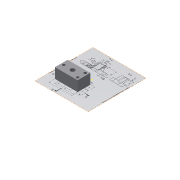
# Autodesk Inventor part: Основание
Saved by Autodesk Inventor 2014 SP1 (Build 180222100, 222)
## iProperties
Created: 2023-10-15
Part Number: Основание
Material: Типовые
Document SubType Name: Modeling
Designer: Konstantin
Density: 1 g/cm^3
Appearance: По умолчанию
Author: Konstantin
Autodesk Inventor part; units mm, degrees
ref_plane "YZ Plane" through (0, 0, 0) normal (1, 0, 0) x (0, 1, 0)
ref_plane "XZ Plane" through (0, 0, 0) normal (0, 1, 0) x (-1, 0, 0)
ref_plane "XY Plane" through (0, 0, 0) normal (0, 0, 1) x (1, 0, 0)
sketch "Эскиз1" plane through (0, 0, 0) normal (0, 0, 1) x (1, 0, 0)
  line L0 (-109.4005, 113.4321) -> (101.5019, 113.4321) construction
  line L1 (101.5019, 113.4321) -> (101.5019, -116.5229) construction
  line L2 (101.5019, -116.5229) -> (-109.4005, -116.5229) construction
  line L3 (-109.4005, -116.5229) -> (-109.4005, 113.4321) construction
  point P0 (0, 0)
  constraints: 2 other
sketch "Эскиз3" plane through (0, 0, 0) normal (0, 0, 1) x (1, 0, 0)
  line L0 (13.0914, -19.0842) -> (-76.7694, -19.0842)
  line L1 (-76.7694, -19.0842) -> (-76.7694, -69.3185)
  line L2 (-76.7694, -69.3185) -> (13.0914, -69.3185)
  line L3 (13.0914, -69.3185) -> (13.0914, -19.0842)
  circle A0 centre (-31.9077, -44.3035) radius 8.6947
  circle A1 centre (-31.9077, -44.3035) radius 14.858
  circle A2 centre (-66.8024, -44.2775) radius 5.0913
  circle A3 centre (3.2723, -59.1355) radius 4.9697
  circle A4 centre (3.2723, -29.4194) radius 5.2903
  line L4 (-61.7111, -29.3433) -> (-64.4086, -29.3433) construction
  line L5 (-64.4086, -29.3433) -> (-66.8024, -30.0442) construction
  line L6 (-66.8024, -30.0442) -> (-70.0469, -31.5698) construction
  line L7 (-70.0469, -31.5698) -> (-73.0319, -33.7588) construction
  line L8 (-73.0319, -33.7588) -> (-75.0219, -36.9428) construction
  line L9 (-75.0219, -36.9428) -> (-76.7694, -40.6575) construction
  line L10 (-76.7694, -40.6575) -> (-76.7694, -44.2013) construction
  line L11 (-76.7694, -44.2013) -> (-76.7694, -47.6888) construction
  line L12 (-76.7694, -47.6888) -> (-75.1545, -51.4698) construction
  line L13 (-75.1545, -51.4698) -> (-72.7665, -54.9191) construction
  line L14 (-72.7665, -54.9191) -> (-69.2509, -57.5061) construction
  line L15 (-69.2509, -57.5061) -> (-66.4649, -58.7001) construction
  line L16 (-66.4649, -58.7001) -> (-63.4136, -59.0593) construction
  line L17 (-63.4136, -59.0593) -> (-61.7111, -59.5624) construction
  spline S0 degree 4 poles (-61.7111, -29.3433) (-64.4086, -29.3433) (-66.8024, -30.0442) (-70.0469, -31.5698) (-73.0319, -33.7588) (-75.0219, -36.9428) (-76.7694, -40.6575) (-76.7694, -44.2013) (-76.7694, -47.6888) (-75.1545, -51.4698) (-72.7665, -54.9191) (-69.2509, -57.5061) (-66.4649, -58.7001) (-63.4136, -59.0593) (-61.7111, -59.5624) knots 1 1 1 1 1 2 3 4 5 6 7 8 9 10 11 12 12 12 12 12
  line L18 (-61.7111, -59.5624) -> (-61.7111, -74.6864)
  line L19 (-61.7111, -29.3433) -> (-61.7111, -13.2619)
  line L20 (-61.7111, -13.2619) -> (-82.7829, -13.2619)
  line L21 (-82.7829, -13.2619) -> (-82.7829, -74.6864)
  line L22 (-82.7829, -74.6864) -> (-61.7111, -74.6864)
  line L23 (0.9069, -17.4974) -> (3.1443, -19.2421) construction
  line L24 (3.1443, -19.2421) -> (3.2723, -19.427) construction
  line L25 (3.2723, -19.427) -> (4.9671, -19.427) construction
  line L26 (4.9671, -19.427) -> (6.9505, -20.1638) construction
  line L27 (6.9505, -20.1638) -> (8.5626, -20.9222) construction
  line L28 (8.5626, -20.9222) -> (10.1498, -22.3051) construction
  line L29 (10.1498, -22.3051) -> (11.3609, -23.7137) construction
  line L30 (11.3609, -23.7137) -> (12.2956, -25.2934) construction
  line L31 (12.2956, -25.2934) -> (13.0914, -26.9858) construction
  line L32 (13.0914, -26.9858) -> (16.1389, -44.0503) construction
  line L33 (16.1389, -44.0503) -> (13.0914, -59.6386) construction
  line L34 (13.0914, -59.6386) -> (13.0914, -61.2275) construction
  line L35 (13.0914, -61.2275) -> (12.4731, -63.3199) construction
  line L36 (12.4731, -63.3199) -> (11.3461, -64.8514) construction
  line L37 (11.3461, -64.8514) -> (10.2973, -66.2768) construction
  line L38 (10.2973, -66.2768) -> (8.7533, -67.6316) construction
  line L39 (8.7533, -67.6316) -> (7.3634, -68.5939) construction
  line L40 (7.3634, -68.5939) -> (4.8885, -69.3185) construction
  line L41 (4.8885, -69.3185) -> (3.2723, -70.0088) construction
  line L42 (3.2723, -70.0088) -> (2.887, -71.3126) construction
  line L43 (2.887, -71.3126) -> (31.3831, -71.3126) construction
  line L44 (31.3831, -71.3126) -> (20.1564, -15.836) construction
  line L45 (20.1564, -15.836) -> (1.0706, -16.7541) construction
  spline S1 degree 4 poles (0.9069, -17.4974) (3.1443, -19.2421) (3.2723, -19.427) (4.9671, -19.427) (6.9505, -20.1638) (8.5626, -20.9222) (10.1498, -22.3051) (11.3609, -23.7137) (12.2956, -25.2934) (13.0914, -26.9858) (16.1389, -44.0503) (13.0914, -59.6386) (13.0914, -61.2275) (12.4731, -63.3199) (11.3461, -64.8514) (10.2973, -66.2768) (8.7533, -67.6316) (7.3634, -68.5939) (4.8885, -69.3185) (3.2723, -70.0088) (2.887, -71.3126) (31.3831, -71.3126) (20.1564, -15.836) (1.0706, -16.7541) knots 1 1 1 1 1 2 3 4 5 6 7 8 9 10 11 12 13 14 15 16 17 18 19 20 21 21 21 21 21
  line L46 (-45.8661, -39.2122) -> (-57.0456, -39.2122)
  line L47 (-57.0456, -39.2122) -> (-57.0456, -49.5793)
  line L48 (-57.0456, -49.5793) -> (-45.7975, -49.5793)
  line L49 (-17.9102, -39.3206) -> (-6.8439, -39.3206)
  line L50 (-6.8439, -39.3206) -> (-6.8439, -49.3593)
  line L51 (-6.8439, -49.3593) -> (-17.9363, -49.3593)
  point P0 (0, 0)
  constraints: 30 end point, 13 perpendicular, 12 parallel, 6 point on line, 5 centre point, 4 point on circle, 1 coincident, 1 collinear, 1 horizontal, 1 midpoint, 6 other
extrude "Выдавливание1" add sketch "Эскиз3" along normal blind 40 contours L3 S1 L0 | S1 L3 L0 | S1 L3 L2 L18 S0 L19 L0 | S1 L3 L2 | L19 S0 L18 L2 L1 L0 | A1 | A1 L49 L50 L51 | A1 L48 L47 L46 picked at (11.6912, -66.5985)
